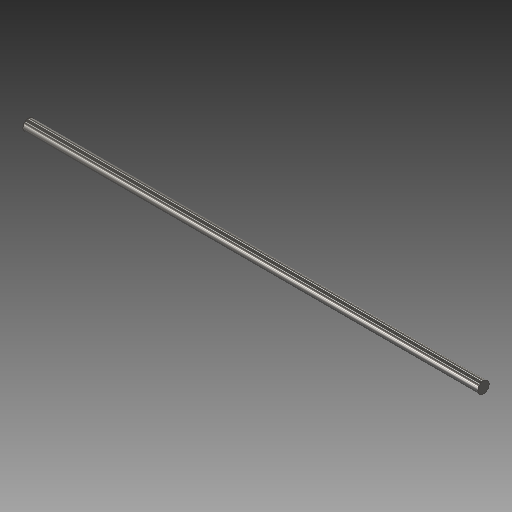
# Autodesk Inventor part: SteelRodForShooter
Saved by Autodesk Inventor 2017 (Build 210142000, 142)
## iProperties
Created: 2016-02-07
Part Number: SteelRodForShooter
Material: Steel, High Strength, Low Alloy
Document SubType Name: Modeling
Designer: steele
Density: 7.85 g/cm^3
Appearance: Steel - Polished
Mass: 184.7 g
Surface Area: 100.233 cm^2
Volume: 23.5286 cm^3
Author: steele
Autodesk Inventor part; units mm, degrees
ref_plane "YZ Plane" through (0, 0, 0) normal (1, 0, 0) x (0, 1, 0)
ref_plane "XZ Plane" through (0, 0, 0) normal (0, 1, 0) x (-1, 0, 0)
ref_plane "XY Plane" through (0, 0, 0) normal (0, 0, 1) x (1, 0, 0)
sketch "Sketch2" plane through (0, 0, 0) normal (1, 0, 0) x (0, 1, 0)
  circle A0 centre (0, 0) radius 4.7625
  dimension "d1" = 9.525
  constraints: 1 centre point, 1 coincident
  measures "d1" diameter of A0
extrude "Extrusion1" add sketch "Sketch2" along normal mid plane 381
equation "\"d1\" = axelDiam"
equation "\"d2\" = axelLength"
equation "\"axelDiam\" = 9.525"
equation "\"axelLength\" = 381"
body "Solid1"
